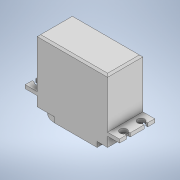
# Autodesk Inventor part: Сервопривод
Saved by Autodesk Inventor 2022 (Build 260153000, 153)
## iProperties
Created: 2022-07-09
Part Number: Сервопривод
Material: Типовые
Document SubType Name: Modeling
Designer: Константин
Density: 1 g/cm^3
Appearance: По умолчанию
Author: Константин
Autodesk Inventor part; units mm, degrees
ref_plane "YZ Plane" through (0, 0, 0) normal (1, 0, 0) x (0, 1, 0)
sketch "Эскиз1" plane through (0, 0, 0) normal (0, 0, 1) x (1, 0, 0)
  line L0 (0, 17.0804) -> (20, 17.0804)
  line L1 (0, 24.5911) -> (0, -44.9718)
  line L2 (14, -21.4196) -> (0, -21.4196)
  line L3 (20, 17.0804) -> (20, -10.9196)
  line L4 (20, -10.9196) -> (26.75, -10.9196)
  line L5 (26.75, -10.9196) -> (26.75, -12.9196)
  line L6 (26.75, -12.9196) -> (20, -12.9196)
  line L7 (20, -12.9196) -> (20, -18.4196)
  line L8 (14, -21.4196) -> (14, -18.4196)
  line L9 (14, -18.4196) -> (20, -18.4196)
  line L10 (0, 17.0804) -> (-20, 17.0804)
  line L11 (-14, -21.4196) -> (0, -21.4196)
  line L12 (-20, 17.0804) -> (-20, -10.9196)
  line L13 (-20, -10.9196) -> (-26.75, -10.9196)
  line L14 (-26.75, -10.9196) -> (-26.75, -12.9196)
  line L15 (-26.75, -12.9196) -> (-20, -12.9196)
  line L16 (-20, -12.9196) -> (-20, -18.4196)
  line L17 (-14, -21.4196) -> (-20, -21.4196)
  line L18 (-20, -21.4196) -> (-20, -18.4196)
  point P0 (0, 0)
  dimension "d14" = 28
  dimension "d15" = 6.75
  dimension "d16" = 2
  dimension "d17" = 6
  dimension "d18" = 3
  dimension "d20" = 20
  constraints: 38 end point, 7 symmetric about line, 6 perpendicular, 4 vertical, 3 horizontal, 2 point on line
  measures "d14" distance of L0.end L3.end
  measures "d15" distance of L3.end L4.end
  measures "d16" distance of L4.end L5.end
  measures "d17" distance of L7.end L8.end
  measures "d18" distance of L2.start L8.end
  measures "d20" distance of L0.start L0.end
extrude "Выдавливание1" add sketch "Эскиз1" along normal blind 20
sketch "Эскиз2" plane through (20, -10.9196, 0) normal (0, 1, 0) x (1, 0, 0)
  line L0 (0, 0) -> (0, -20) projected
  line L1 (0, -10) -> (9.888, -10)
  arc A0 (5.7321, -4) -> (5.7321, -6) centre (4, -5) ccw
  line L2 (6.75, 0) -> (6.75, -20) projected
  line L3 (6, -4) -> (6.75, -4)
  line L4 (6, -6) -> (6.75, -6)
  line L5 (6, -4) -> (5.7321, -4)
  line L6 (6, -6) -> (5.7321, -6)
  point P0 (-20, 0)
  dimension "d23" = 4
  dimension "d24" = 3
  dimension "d25" = 2
  constraints: 10 end point, 4 horizontal, 2 point on circle, 1 centre point, 1 midpoint, 3 other
  measures "d23" diameter of A0
  measures "d24" distance edge to line of A0 L1
  measures "d25" distance edge to line of A0 L0
extrude "Выдавливание2" cut sketch "Эскиз2" against normal through all
ref_plane "РабПлоскость1" through (0, 0, 10) normal (0, 0, 1) x (1, 0, 0)
mirror "Зеркальное отражение2" about plane through (0, 0, 10) normal (0, 0, 1) of "Выдавливание2"
ref_plane "РабПлоскость3" through (0, -10.9196, 0) normal (1, 0, 0) x (0, 0, -1)
mirror "Зеркальное отражение3" about plane through (0, -10.9196, 0) normal (1, 0, 0) of "Выдавливание2", "Зеркальное отражение2"
chamfer "Фаска1" distance 1 angle 45 4 edges at (0, 17.0804, 20) (20, 17.0804, 10) (0, 17.0804, 0) (-20, 17.0804, 10)
sketch "Эскиз3" plane through (-14, -21.4196, 0) normal (0, -1, 0) x (1, 0, 0)
  line L0 (28, 0) -> (28, 20) projected
  line L1 (-6, 0) -> (-6, 20)
  line L2 (-6, 20) -> (34, 20) projected
  circle A0 centre (4, 10) radius 10
  circle A1 centre (4, 10) radius 2.75
  circle A2 centre (4, 10) radius 5.25
  circle A3 centre (4, 10) radius 6.5
  line L3 (-6, 0) -> (-12.75, 0) projected
  line L4 (-6, 0) -> (4, 0)
  line L5 (-6, 20) -> (4, 20)
  line L6 (-6, 20) -> (28, 20) projected
  line L7 (-6, 0) -> (-6, 20) projected
  line L8 (-6, 0) -> (-6, 20)
  point P0 (14, 0)
  point P1 (-6, 10)
  dimension "d39" = 5.5
  dimension "d41" = 10.5
  dimension "d42" = 13
  constraints: 8 end point, 4 centre point, 3 coincident, 2 point on circle, 1 point on line, 1 tangent, 1 vertical
  measures "d39" diameter of A1
  measures "d41" diameter of A2
  measures "d42" diameter of A3
extrude "Выдавливание3" cut sketch "Эскиз3" against normal up to surface (3 mm away) contours L1 A0 L4 | L1 L2 A0
sketch "Эскиз5" plane through (14, -21.4196, 0) normal (0, -1, 0) x (1, 0, 0)
  point P0 (-14, 0)
extrude "Выдавливание4" add sketch "Эскиз3" along normal blind 1 contours A3
extrude "Выдавливание5" add sketch "Эскиз3" along normal blind 1.5 contours A2
extrude "Выдавливание6" add sketch "Эскиз3" along normal blind 6 contours A1
sketch "Эскиз6" plane through (-10, -27.4196, 10) normal (0, -1, 0) x (1, 0, 0)
  circle A0 centre (0, 0) radius 1
  point P0 (10, -10)
  dimension "d52" = 2
  constraints: 1 centre point
  measures "d52" diameter of A0
extrude "Выдавливание7" cut sketch "Эскиз6" against normal up to surface (9 mm away)
